phone-robot-case-v1 (Autodesk Fusion 360 design; units mm, degrees)
part number: 2026-09-02-14-29-54-371
part number: 2026-09-02-16-09-22-957
part number: 2026-09-07-14-43-40-851
part number: 2026-09-07-14-43-47-610
Autodesk Fusion 360 part; units mm, degrees
(part 1 of 2)
sketch "スケッチ1" plane through (0, 0, 0) normal (0, 0, 1) x (1, 0, 0) in component "iPhone SE 3 - Parametric Drawing Model"
  arc A0 (33.635, 60.12) -> (24.535, 69.22) centre (24.535, 60.12) ccw
  arc A1 (24.535, -69.22) -> (33.635, -60.12) centre (24.535, -60.12) ccw
  arc A2 (-33.635, -60.12) -> (-24.535, -69.22) centre (-24.535, -60.12) ccw
  arc A3 (-24.535, 69.22) -> (-33.635, 60.12) centre (-24.535, 60.12) ccw
  line L0 (-24.535, 69.22) -> (24.535, 69.22)
  line L1 (33.635, 60.12) -> (33.635, -60.12)
  line L2 (24.535, -69.22) -> (-24.535, -69.22)
  line L3 (-33.635, -60.12) -> (-33.635, 60.12)
  dimension "d710" = 49.07
  dimension "d711" = 120.24
  dimension "d712" = 9.1
  dimension "d713" = 24.535
  dimension "d714" = 60.12
  constraint horizontal L0
  constraint horizontal L2
  constraint vertical L3
  constraint vertical L1
  constraint tangent A0 L0
  constraint tangent A0 L1
  constraint tangent A1 L1
  constraint tangent A1 L2
  constraint tangent A2 L2
  constraint tangent A2 L3
  constraint tangent A3 L3
  constraint tangent A3 L0
  constraint equal A0 A1
  constraint equal A0 A2
  constraint equal A0 A3
  measures "d710" horizontal distance of A0.end A3.start
  measures "d711" vertical distance of A0.start A1.end
  measures "d712" radius of A0
  measures "d713" horizontal distance of origin A0.centre
  measures "d714" vertical distance of origin A0.centre
extrude "Rear Glass" add sketch "スケッチ1" along normal blind 0.9 makes body 1 in component "iPhone SE 3 - Parametric Drawing Model"
ref_plane "作業平面1" through (0, 0, 0.9) normal (0, 0, 1) x (1, 0, 0) in component "iPhone SE 3 - Parametric Drawing Model"
sketch "スケッチ2" plane through (0, 0, 0.9) normal (0, 0, 1) x (1, 0, 0) in component "iPhone SE 3 - Parametric Drawing Model"
  arc A0 (33.635, 60.12) -> (24.535, 69.22) centre (24.535, 60.12) ccw
  arc A1 (24.535, -69.22) -> (33.635, -60.12) centre (24.535, -60.12) ccw
  arc A2 (-33.635, -60.12) -> (-24.535, -69.22) centre (-24.535, -60.12) ccw
  arc A3 (-24.535, 69.22) -> (-33.635, 60.12) centre (-24.535, 60.12) ccw
  line L0 (-24.535, 69.22) -> (24.535, 69.22)
  line L1 (33.635, 60.12) -> (33.635, -60.12)
  line L2 (24.535, -69.22) -> (-24.535, -69.22)
  line L3 (-33.635, -60.12) -> (-33.635, 60.12)
  dimension "d719" = 49.07
  dimension "d720" = 120.24
  dimension "d721" = 9.1
  dimension "d722" = 24.535
  dimension "d723" = 60.12
  constraint horizontal L0
  constraint horizontal L2
  constraint vertical L3
  constraint vertical L1
  constraint tangent A0 L0
  constraint tangent A0 L1
  constraint tangent A1 L1
  constraint tangent A1 L2
  constraint tangent A2 L2
  constraint tangent A2 L3
  constraint tangent A3 L3
  constraint tangent A3 L0
  constraint equal A0 A1
  constraint equal A0 A2
  constraint equal A0 A3
  measures "d719" horizontal distance of A0.end A3.start
  measures "d720" vertical distance of A0.start A1.end
  measures "d721" radius of A0
  measures "d722" horizontal distance of origin A0.centre
  measures "d723" vertical distance of origin A0.centre
extrude "Aluminum Frame" add sketch "スケッチ2" along normal blind 5.51 separate body makes body 2 in component "iPhone SE 3 - Parametric Drawing Model"
ref_plane "作業平面2" through (0, 0, 6.41) normal (0, 0, 1) x (1, 0, 0) in component "iPhone SE 3 - Parametric Drawing Model"
sketch "スケッチ3" plane through (0, 0, 6.41) normal (0, 0, 1) x (1, 0, 0) in component "iPhone SE 3 - Parametric Drawing Model"
  arc A0 (33.635, 60.12) -> (24.535, 69.22) centre (24.535, 60.12) ccw
  arc A1 (24.535, -69.22) -> (33.635, -60.12) centre (24.535, -60.12) ccw
  arc A2 (-33.635, -60.12) -> (-24.535, -69.22) centre (-24.535, -60.12) ccw
  arc A3 (-24.535, 69.22) -> (-33.635, 60.12) centre (-24.535, 60.12) ccw
  line L0 (-24.535, 69.22) -> (24.535, 69.22)
  line L1 (33.635, 60.12) -> (33.635, -60.12)
  line L2 (24.535, -69.22) -> (-24.535, -69.22)
  line L3 (-33.635, -60.12) -> (-33.635, 60.12)
  dimension "d728" = 49.07
  dimension "d729" = 120.24
  dimension "d730" = 9.1
  dimension "d731" = 24.535
  dimension "d732" = 60.12
  constraint horizontal L0
  constraint horizontal L2
  constraint vertical L3
  constraint vertical L1
  constraint tangent A0 L0
  constraint tangent A0 L1
  constraint tangent A1 L1
  constraint tangent A1 L2
  constraint tangent A2 L2
  constraint tangent A2 L3
  constraint tangent A3 L3
  constraint tangent A3 L0
  constraint equal A0 A1
  constraint equal A0 A2
  constraint equal A0 A3
  measures "d728" horizontal distance of A0.end A3.start
  measures "d729" vertical distance of A0.start A1.end
  measures "d730" radius of A0
  measures "d731" horizontal distance of origin A0.centre
  measures "d732" vertical distance of origin A0.centre
extrude "Front Cover Glass" add sketch "スケッチ3" along normal blind 0.9 separate body makes body 3 in component "iPhone SE 3 - Parametric Drawing Model"
ref_plane "作業平面3" through (0, 0, 7.31) normal (0, 0, 1) x (1, 0, 0) in component "iPhone SE 3 - Parametric Drawing Model"
sketch "スケッチ4" plane through (0, 0, 7.31) normal (0, 0, 1) x (1, 0, 0) in component "iPhone SE 3 - Parametric Drawing Model"
  arc A0 (29.25, 51.23) -> (28.45, 52.03) centre (28.45, 51.23) ccw
  arc A1 (28.45, -52.02) -> (29.25, -51.22) centre (28.45, -51.22) ccw
  arc A2 (-29.25, -51.22) -> (-28.45, -52.02) centre (-28.45, -51.22) ccw
  arc A3 (-28.45, 52.03) -> (-29.25, 51.23) centre (-28.45, 51.23) ccw
  line L0 (-28.45, 52.03) -> (28.45, 52.03)
  line L1 (29.25, 51.23) -> (29.25, -51.22)
  line L2 (28.45, -52.02) -> (-28.45, -52.02)
  line L3 (-29.25, -51.22) -> (-29.25, 51.23)
  dimension "d737" = 56.9
  dimension "d738" = 102.45
  dimension "d739" = 0.8
  dimension "d740" = 28.45
  dimension "d741" = 51.23
  constraint horizontal L0
  constraint horizontal L2
  constraint vertical L3
  constraint vertical L1
  constraint tangent A0 L0
  constraint tangent A0 L1
  constraint tangent A1 L1
  constraint tangent A1 L2
  constraint tangent A2 L2
  constraint tangent A2 L3
  constraint tangent A3 L3
  constraint tangent A3 L0
  constraint equal A0 A1
  constraint equal A0 A2
  constraint equal A0 A3
  measures "d737" horizontal distance of A0.end A3.start
  measures "d738" vertical distance of A0.start A1.end
  measures "d739" radius of A0
  measures "d740" horizontal distance of origin A0.centre
  measures "d741" vertical distance of origin A0.centre
extrude "Front Active Area Reference" add sketch "スケッチ4" along normal blind 0.02 separate body makes body 4 in component "iPhone SE 3 - Parametric Drawing Model"
sketch "スケッチ5" plane through (0, 0, 7.31) normal (0, 0, 1) x (1, 0, 0) in component "iPhone SE 3 - Parametric Drawing Model"
  circle A0 centre (0, -59.97) radius 5.45
  dimension "d744" = 59.97
  dimension "d745" = 10.9
  constraint vertical origin A0.centre
  measures "d744" vertical distance of origin A0.centre
  measures "d745" diameter of A0
extrude "Home Touch ID Sensor" add sketch "スケッチ5" along normal blind 0.02 separate body makes body 5 in component "iPhone SE 3 - Parametric Drawing Model"
sketch "スケッチ6" plane through (0, 0, 7.31) normal (0, 0, 1) x (1, 0, 0) in component "iPhone SE 3 - Parametric Drawing Model"
  circle A0 centre (-10.645, 60.12) radius 1.605
  dimension "d748" = 10.645
  dimension "d749" = 60.12
  dimension "d750" = 3.21
  measures "d748" horizontal distance of origin A0.centre
  measures "d749" vertical distance of origin A0.centre
  measures "d750" diameter of A0
extrude "Front Detail 12 Front Camera Position" add sketch "スケッチ6" along normal blind 0.02 separate body makes body 6 in component "iPhone SE 3 - Parametric Drawing Model"
sketch "スケッチ7" plane through (0, 0, 7.31) normal (0, 0, 1) x (1, 0, 0) in component "iPhone SE 3 - Parametric Drawing Model"
  circle A0 centre (-0.005, 64.38) radius 1
  dimension "d753" = 0.005
  dimension "d754" = 64.38
  dimension "d755" = 2
  measures "d753" horizontal distance of origin A0.centre
  measures "d754" vertical distance of origin A0.centre
  measures "d755" diameter of A0
extrude "Front Detail 13 Proximity Sensor Position" add sketch "スケッチ7" along normal blind 0.02 separate body makes body 7 in component "iPhone SE 3 - Parametric Drawing Model"
sketch "スケッチ8" plane through (0, 0, 7.31) normal (0, 0, 1) x (1, 0, 0) in component "iPhone SE 3 - Parametric Drawing Model"
  circle A0 centre (3.685, 64.38) radius 1
  dimension "d758" = 3.685
  dimension "d759" = 64.38
  dimension "d760" = 2
  measures "d758" horizontal distance of origin A0.centre
  measures "d759" vertical distance of origin A0.centre
  measures "d760" diameter of A0
extrude "Front Detail 14 ALS Position" add sketch "スケッチ8" along normal blind 0.02 separate body makes body 8 in component "iPhone SE 3 - Parametric Drawing Model"
sketch "スケッチ9" plane through (0, 0, 7.31) normal (0, 0, 1) x (1, 0, 0) in component "iPhone SE 3 - Parametric Drawing Model"
  arc A0 (5.335, 59.52) -> (5.335, 60.72) centre (5.335, 60.12) ccw
  arc A1 (-5.335, 60.72) -> (-5.335, 59.52) centre (-5.335, 60.12) ccw
  line L0 (-5.335, 60.72) -> (5.335, 60.72)
  line L1 (5.335, 59.52) -> (-5.335, 59.52)
  line L2 (-5.335, 60.12) -> (5.335, 60.12) construction
  point P0 (0, 60.12)
  dimension "d763" = 10.67
  dimension "d764" = 0.6
  dimension "d765" = 60.12
  constraint horizontal L0
  constraint horizontal L1
  constraint equal A0 A1
  constraint midpoint L2 P0
  constraint vertical origin P0
  measures "d763" horizontal distance of A0.centre A1.centre
  measures "d764" radius of A0
  measures "d765" vertical distance of origin P0
extrude "Receiver Opening" add sketch "スケッチ9" along normal blind 0.02 separate body makes body 9 in component "iPhone SE 3 - Parametric Drawing Model"
sketch "スケッチ10" plane through (0, 0, 0) normal (0, 0, 1) x (1, 0, 0) in component "iPhone SE 3 - Parametric Drawing Model"
  circle A0 centre (-23.195, 53.82) radius 4.285
  dimension "d768" = 23.195
  dimension "d769" = 53.82
  dimension "d770" = 8.57
  measures "d768" horizontal distance of origin A0.centre
  measures "d769" vertical distance of origin A0.centre
  measures "d770" diameter of A0
extrude "Rear Camera Bump" add sketch "スケッチ10" against normal blind 0.87 separate body makes body 10 in component "iPhone SE 3 - Parametric Drawing Model"
sketch "スケッチ11" plane through (0, 0, 0) normal (0, 0, 1) x (1, 0, 0) in component "iPhone SE 3 - Parametric Drawing Model"
  circle A0 centre (-15.505, 53.82) radius 0.75
  dimension "d773" = 15.505
  dimension "d774" = 53.82
  dimension "d775" = 1.5
  measures "d773" horizontal distance of origin A0.centre
  measures "d774" vertical distance of origin A0.centre
  measures "d775" diameter of A0
extrude "Rear Microphone" add sketch "スケッチ11" against normal blind 0.02 separate body makes body 11 in component "iPhone SE 3 - Parametric Drawing Model"
sketch "スケッチ12" plane through (0, 0, 0) normal (0, 0, 1) x (1, 0, 0) in component "iPhone SE 3 - Parametric Drawing Model"
  circle A0 centre (-10.795, 53.82) radius 1.875
  dimension "d778" = 10.795
  dimension "d779" = 53.82
  dimension "d780" = 3.75
  measures "d778" horizontal distance of origin A0.centre
  measures "d779" vertical distance of origin A0.centre
  measures "d780" diameter of A0
extrude "Rear Flash" add sketch "スケッチ12" against normal blind 0.02 separate body makes body 12 in component "iPhone SE 3 - Parametric Drawing Model"
ref_plane "作業平面4" through (-33.635, 0, 0) normal (1, 0, 0) x (0, 1, 0) in component "iPhone SE 3 - Parametric Drawing Model"
ref_plane "作業平面5" through (33.635, 0, 0) normal (1, 0, 0) x (0, 1, 0) in component "iPhone SE 3 - Parametric Drawing Model"
sketch "スケッチ13" plane through (-33.635, 0, 0) normal (1, 0, 0) x (0, 0, -1) in component "iPhone SE 3 - Parametric Drawing Model"
  arc A0 (-2.755, 50.76) -> (-4.555, 50.76) centre (-3.655, 50.76) ccw
  arc A1 (-4.555, 46.95) -> (-2.755, 46.95) centre (-3.655, 46.95) ccw
  line L0 (-2.755, 50.76) -> (-2.755, 46.95)
  line L1 (-4.555, 46.95) -> (-4.555, 50.76)
  line L2 (-3.655, 50.76) -> (-3.655, 46.95) construction
  point P0 (-3.655, 48.855)
  dimension "d787" = 3.81
  dimension "d788" = 0.9
  dimension "d789" = 3.655
  dimension "d790" = 48.855
  constraint vertical L0
  constraint vertical L1
  constraint equal A0 A1
  constraint midpoint L2 P0
  measures "d787" vertical distance of A0.centre A1.centre
  measures "d788" radius of A0
  measures "d789" horizontal distance of origin P0
  measures "d790" vertical distance of origin P0
extrude "Ring Silent Switch" add sketch "スケッチ13" against normal blind 0.42 separate body makes body 13 in component "iPhone SE 3 - Parametric Drawing Model"
sketch "スケッチ14" plane through (-33.635, 0, 0) normal (1, 0, 0) x (0, 0, -1) in component "iPhone SE 3 - Parametric Drawing Model"
  arc A0 (-2.755, 39.07) -> (-4.555, 39.07) centre (-3.655, 39.07) ccw
  arc A1 (-4.555, 30.25) -> (-2.755, 30.25) centre (-3.655, 30.25) ccw
  line L0 (-2.755, 39.07) -> (-2.755, 30.25)
  line L1 (-4.555, 30.25) -> (-4.555, 39.07)
  line L2 (-3.655, 39.07) -> (-3.655, 30.25) construction
  point P0 (-3.655, 34.66)
  dimension "d793" = 8.82
  dimension "d794" = 0.9
  dimension "d795" = 3.655
  dimension "d796" = 34.66
  constraint vertical L0
  constraint vertical L1
  constraint equal A0 A1
  constraint midpoint L2 P0
  measures "d793" vertical distance of A0.centre A1.centre
  measures "d794" radius of A0
  measures "d795" horizontal distance of origin P0
  measures "d796" vertical distance of origin P0
extrude "Volume Plus Button" add sketch "スケッチ14" against normal blind 0.4 separate body makes body 14 in component "iPhone SE 3 - Parametric Drawing Model"
sketch "スケッチ15" plane through (-33.635, 0, 0) normal (1, 0, 0) x (0, 0, -1) in component "iPhone SE 3 - Parametric Drawing Model"
  arc A0 (-2.755, 26.46) -> (-4.555, 26.46) centre (-3.655, 26.46) ccw
  arc A1 (-4.555, 17.64) -> (-2.755, 17.64) centre (-3.655, 17.64) ccw
  line L0 (-2.755, 26.46) -> (-2.755, 17.64)
  line L1 (-4.555, 17.64) -> (-4.555, 26.46)
  line L2 (-3.655, 26.46) -> (-3.655, 17.64) construction
  point P0 (-3.655, 22.05)
  dimension "d799" = 8.82
  dimension "d800" = 0.9
  dimension "d801" = 3.655
  dimension "d802" = 22.05
  constraint vertical L0
  constraint vertical L1
  constraint equal A0 A1
  constraint midpoint L2 P0
  measures "d799" vertical distance of A0.centre A1.centre
  measures "d800" radius of A0
  measures "d801" horizontal distance of origin P0
  measures "d802" vertical distance of origin P0
extrude "Volume Minus Button" add sketch "スケッチ15" against normal blind 0.4 separate body makes body 15 in component "iPhone SE 3 - Parametric Drawing Model"
sketch "スケッチ16" plane through (33.635, 0, 0) normal (1, 0, 0) x (0, 0, -1) in component "iPhone SE 3 - Parametric Drawing Model"
  arc A0 (-2.755, 38.99) -> (-4.555, 38.99) centre (-3.655, 38.99) ccw
  arc A1 (-4.555, 30.17) -> (-2.755, 30.17) centre (-3.655, 30.17) ccw
  line L0 (-2.755, 38.99) -> (-2.755, 30.17)
  line L1 (-4.555, 30.17) -> (-4.555, 38.99)
  line L2 (-3.655, 38.99) -> (-3.655, 30.17) construction
  point P0 (-3.655, 34.58)
  dimension "d805" = 8.82
  dimension "d806" = 0.9
  dimension "d807" = 3.655
  dimension "d808" = 34.58
  constraint vertical L0
  constraint vertical L1
  constraint equal A0 A1
  constraint midpoint L2 P0
  measures "d805" vertical distance of A0.centre A1.centre
  measures "d806" radius of A0
  measures "d807" horizontal distance of origin P0
  measures "d808" vertical distance of origin P0
extrude "Side Button" add sketch "スケッチ16" along normal blind 0.4 separate body makes body 16 in component "iPhone SE 3 - Parametric Drawing Model"
sketch "スケッチ17" plane through (33.635, 0, 0) normal (1, 0, 0) x (0, 0, -1) in component "iPhone SE 3 - Parametric Drawing Model"
  arc A0 (-2.505, 15.35) -> (-4.805, 15.35) centre (-3.655, 15.35) ccw
  arc A1 (-4.805, 1.98) -> (-2.505, 1.98) centre (-3.655, 1.98) ccw
  line L0 (-2.505, 15.35) -> (-2.505, 1.98)
  line L1 (-4.805, 1.98) -> (-4.805, 15.35)
  line L2 (-3.655, 15.35) -> (-3.655, 1.98) construction
  point P0 (-3.655, 8.665)
  dimension "d811" = 13.37
  dimension "d812" = 1.15
  dimension "d813" = 3.655
  dimension "d814" = 8.665
  constraint vertical L0
  constraint vertical L1
  constraint equal A0 A1
  constraint midpoint L2 P0
  measures "d811" vertical distance of A0.centre A1.centre
  measures "d812" radius of A0
  measures "d813" horizontal distance of origin P0
  measures "d814" vertical distance of origin P0
extrude "SIM Tray Seam" cut sketch "スケッチ17" against normal blind 0.05 bodies 2 in component "iPhone SE 3 - Parametric Drawing Model"
ref_plane "作業平面6" through (0, -69.22, 0) normal (0, 1, 0) x (0, 0, 1) in component "iPhone SE 3 - Parametric Drawing Model"
sketch "スケッチ18" plane through (0, -69.22, 0) normal (0, 1, 0) x (1, 0, 0) in component "iPhone SE 3 - Parametric Drawing Model"
  arc A0 (3.55, -4.455) -> (3.55, -2.855) centre (3.55, -3.655) ccw
  arc A1 (-3.55, -2.855) -> (-3.55, -4.455) centre (-3.55, -3.655) ccw
  line L0 (-3.55, -2.855) -> (3.55, -2.855)
  line L1 (3.55, -4.455) -> (-3.55, -4.455)
  line L2 (-3.55, -3.655) -> (3.55, -3.655) construction
  circle A2 centre (-23.375, -3.655) radius 0.725
  circle A3 centre (-20.975, -3.655) radius 0.725
  circle A4 centre (-18.575, -3.655) radius 0.725
  circle A5 centre (-16.175, -3.655) radius 0.725
  circle A6 centre (-13.775, -3.655) radius 0.725
  circle A7 centre (-11.375, -3.655) radius 0.725
  circle A8 centre (11.375, -3.655) radius 0.725
  circle A9 centre (13.775, -3.655) radius 0.725
  circle A10 centre (16.175, -3.655) radius 0.725
  circle A11 centre (18.575, -3.655) radius 0.725
  circle A12 centre (20.975, -3.655) radius 0.725
  circle A13 centre (23.375, -3.655) radius 0.725
  circle A14 centre (-6.395, -3.655) radius 0.8
  circle A15 centre (6.395, -3.655) radius 0.8
  point P0 (0, -3.655)
  dimension "d819" = 7.1
  dimension "d820" = 0.8
  dimension "d821" = 3.655
  dimension "d822" = 23.375
  dimension "d823" = 3.655
  dimension "d824" = 1.45
  dimension "d825" = 20.975
  dimension "d826" = 3.655
  dimension "d827" = 1.45
  dimension "d828" = 18.575
  dimension "d829" = 3.655
  dimension "d830" = 1.45
  dimension "d831" = 16.175
  dimension "d832" = 3.655
  dimension "d833" = 1.45
  dimension "d834" = 13.775
  dimension "d835" = 3.655
  dimension "d836" = 1.45
  dimension "d837" = 11.375
  dimension "d838" = 3.655
  dimension "d839" = 1.45
  dimension "d840" = 11.375
  dimension "d841" = 3.655
  dimension "d842" = 1.45
  dimension "d843" = 13.775
  dimension "d844" = 3.655
  dimension "d845" = 1.45
  dimension "d846" = 16.175
  dimension "d847" = 3.655
  dimension "d848" = 1.45
  dimension "d849" = 18.575
  dimension "d850" = 3.655
  dimension "d851" = 1.45
  dimension "d852" = 20.975
  dimension "d853" = 3.655
  dimension "d854" = 1.45
  dimension "d855" = 23.375
  dimension "d856" = 3.655
  dimension "d857" = 1.45
  dimension "d858" = 6.395
  dimension "d859" = 3.655
  dimension "d860" = 1.6
  dimension "d861" = 6.395
  dimension "d862" = 3.655
  dimension "d863" = 1.6
  constraint horizontal L0
  constraint horizontal L1
  constraint equal A0 A1
  constraint midpoint L2 P0
  constraint vertical origin P0
  measures "d819" horizontal distance of A0.centre A1.centre
  measures "d820" radius of A0
  measures "d821" vertical distance of origin P0
  measures "d822" horizontal distance of origin A2.centre
  measures "d823" vertical distance of origin A2.centre
  measures "d824" diameter of A2
  measures "d825" horizontal distance of origin A3.centre
  measures "d826" vertical distance of origin A3.centre
  measures "d827" diameter of A3
  measures "d828" horizontal distance of origin A4.centre
  measures "d829" vertical distance of origin A4.centre
  measures "d830" diameter of A4
  measures "d831" horizontal distance of origin A5.centre
  measures "d832" vertical distance of origin A5.centre
  measures "d833" diameter of A5
  measures "d834" horizontal distance of origin A6.centre
  measures "d835" vertical distance of origin A6.centre
  measures "d836" diameter of A6
  measures "d837" horizontal distance of origin A7.centre
  measures "d838" vertical distance of origin A7.centre
  measures "d839" diameter of A7
  measures "d840" horizontal distance of origin A8.centre
  measures "d841" vertical distance of origin A8.centre
  measures "d842" diameter of A8
  measures "d843" horizontal distance of origin A9.centre
  measures "d844" vertical distance of origin A9.centre
  measures "d845" diameter of A9
  measures "d846" horizontal distance of origin A10.centre
  measures "d847" vertical distance of origin A10.centre
  measures "d848" diameter of A10
  measures "d849" horizontal distance of origin A11.centre
  measures "d850" vertical distance of origin A11.centre
  measures "d851" diameter of A11
  measures "d852" horizontal distance of origin A12.centre
  measures "d853" vertical distance of origin A12.centre
  measures "d854" diameter of A12
  measures "d855" horizontal distance of origin A13.centre
  measures "d856" vertical distance of origin A13.centre
  measures "d857" diameter of A13
  measures "d858" horizontal distance of origin A14.centre
  measures "d859" vertical distance of origin A14.centre
  measures "d860" diameter of A14
  measures "d861" horizontal distance of origin A15.centre
  measures "d862" vertical distance of origin A15.centre
  measures "d863" diameter of A15
extrude "Bottom Port and Acoustic Openings" cut sketch "スケッチ18" along normal blind 1 bodies 2 in component "iPhone SE 3 - Parametric Drawing Model"
ref_plane "作業平面7" through (0, 0, 3.655) normal (0, 0, 1) x (1, 0, 0) in component "iPhone SE 3 - Parametric Drawing Model"
sketch "スケッチ19" plane through (0, 0, 3.655) normal (0, 0, 1) x (1, 0, 0) in component "iPhone SE 3 - Parametric Drawing Model"
  arc A0 (33.635, 60.12) -> (24.535, 69.22) centre (24.535, 60.12) ccw
  arc A1 (24.535, -69.22) -> (33.635, -60.12) centre (24.535, -60.12) ccw
  arc A2 (-33.635, -60.12) -> (-24.535, -69.22) centre (-24.535, -60.12) ccw
  arc A3 (-24.535, 69.22) -> (-33.635, 60.12) centre (-24.535, 60.12) ccw
  line L0 (-24.535, 69.22) -> (24.535, 69.22)
  line L1 (33.635, 60.12) -> (33.635, -60.12)
  line L2 (24.535, -69.22) -> (-24.535, -69.22)
  line L3 (-33.635, -60.12) -> (-33.635, 60.12)
  dimension "d868" = 49.07
  dimension "d869" = 120.24
  dimension "d870" = 9.1
  dimension "d871" = 24.535
  dimension "d872" = 60.12
  constraint horizontal L0
  constraint horizontal L2
  constraint vertical L3
  constraint vertical L1
  constraint tangent A0 L0
  constraint tangent A0 L1
  constraint tangent A1 L1
  constraint tangent A1 L2
  constraint tangent A2 L2
  constraint tangent A2 L3
  constraint tangent A3 L3
  constraint tangent A3 L0
  constraint equal A0 A1
  constraint equal A0 A2
  constraint equal A0 A3
  measures "d868" horizontal distance of A0.end A3.start
  measures "d869" vertical distance of A0.start A1.end
  measures "d870" radius of A0
  measures "d871" horizontal distance of origin A0.centre
  measures "d872" vertical distance of origin A0.centre
ref_plane "作業平面1" through (0, 0, -2.9) normal (0, 0, 1) x (1, 0, 0) in component "Robot V1 - A Holder and Stand"
ref_plane "作業平面2" through (0, 0, -0.5) normal (0, 0, 1) x (1, 0, 0) in component "Robot V1 - A Holder and Stand"
ref_plane "作業平面3" through (0, 0, 7.71) normal (0, 0, 1) x (1, 0, 0) in component "Robot V1 - A Holder and Stand"
sketch "スケッチ1 (2)" plane through (0, 0, -2.9) normal (0, 0, 1) x (1, 0, 0) in component "Robot V1 - A Holder and Stand"
  arc A0 (46, 68) -> (40, 74) centre (40, 68) ccw
  arc A1 (40, 14) -> (46, 20) centre (40, 20) ccw
  arc A2 (-46, 20) -> (-40, 14) centre (-40, 20) ccw
  arc A3 (-40, 74) -> (-46, 68) centre (-40, 68) ccw
  line L0 (-40, 74) -> (40, 74)
  line L1 (46, 68) -> (46, 20)
  line L2 (40, 14) -> (-40, 14)
  line L3 (-46, 20) -> (-46, 68)
  line L4 (40, 68) -> (-40, 20) construction
  point P0 (0, 44)
  dimension "d1520" = 80
  dimension "d1521" = 48
  dimension "d1522" = 6
  dimension "d1523" = 44
  constraint horizontal L0
  constraint horizontal L2
  constraint vertical L3
  constraint vertical L1
  constraint tangent A0 L0
  constraint tangent A0 L1
  constraint tangent A1 L1
  constraint tangent A1 L2
  constraint tangent A2 L2
  constraint tangent A2 L3
  constraint tangent A3 L3
  constraint tangent A3 L0
  constraint equal A0 A1
  constraint equal A0 A2
  constraint equal A0 A3
  constraint midpoint L4 P0
  constraint vertical origin P0
  measures "d1520" horizontal distance of A0.end A3.start
  measures "d1521" vertical distance of A0.start A1.end
  measures "d1522" radius of A0
  measures "d1523" vertical distance of origin P0
extrude "A 01 Head plate" add sketch "スケッチ1 (2)" along normal blind 2.4 separate body makes body 17 in component "Robot V1 - A Holder and Stand"
sketch "スケッチ2 (2)" plane through (0, 0, -2.9) normal (0, 0, 1) x (1, 0, 0) in component "Robot V1 - A Holder and Stand"
  arc A0 (41, 16) -> (35, 22) centre (35, 16) ccw
  arc A1 (35, -74) -> (41, -68) centre (35, -68) ccw
  arc A2 (-41, -68) -> (-35, -74) centre (-35, -68) ccw
  arc A3 (-35, 22) -> (-41, 16) centre (-35, 16) ccw
  line L0 (-35, 22) -> (35, 22)
  line L1 (41, 16) -> (41, -68)
  line L2 (35, -74) -> (-35, -74)
  line L3 (-41, -68) -> (-41, 16)
  line L4 (35, 16) -> (-35, -68) construction
  point P0 (0, -26)
  dimension "d1526" = 70
  dimension "d1527" = 84
  dimension "d1528" = 6
  dimension "d1529" = 26
  constraint horizontal L0
  constraint horizontal L2
  constraint vertical L3
  constraint vertical L1
  constraint tangent A0 L0
  constraint tangent A0 L1
  constraint tangent A1 L1
  constraint tangent A1 L2
  constraint tangent A2 L2
  constraint tangent A2 L3
  constraint tangent A3 L3
  constraint tangent A3 L0
  constraint equal A0 A1
  constraint equal A0 A2
  constraint equal A0 A3
  constraint midpoint L4 P0
  constraint vertical origin P0
  measures "d1526" horizontal distance of A0.end A3.start
  measures "d1527" vertical distance of A0.start A1.end
  measures "d1528" radius of A0
  measures "d1529" vertical distance of origin P0
extrude "A 02 Body plate" add sketch "スケッチ2 (2)" along normal blind 2.4 bodies 17 in component "Robot V1 - A Holder and Stand"
sketch "スケッチ3 (2)" plane through (0, 0, -0.5) normal (0, 0, 1) x (1, 0, 0) in component "Robot V1 - A Holder and Stand"
  arc A0 (36.435, 60.12) -> (24.535, 72.02) centre (24.535, 60.12) ccw
  arc A1 (24.535, -72.02) -> (36.435, -60.12) centre (24.535, -60.12) ccw
  arc A2 (-36.435, -60.12) -> (-24.535, -72.02) centre (-24.535, -60.12) ccw
  arc A3 (-24.535, 72.02) -> (-36.435, 60.12) centre (-24.535, 60.12) ccw
  line L0 (-24.535, 72.02) -> (24.535, 72.02)
  line L1 (36.435, 60.12) -> (36.435, -60.12)
  line L2 (24.535, -72.02) -> (-24.535, -72.02)
  line L3 (-36.435, -60.12) -> (-36.435, 60.12)
  line L4 (24.535, 60.12) -> (-24.535, -60.12) construction
  dimension "d1532" = 49.07
  dimension "d1533" = 120.24
  dimension "d1534" = 11.9
  constraint horizontal L0
  constraint horizontal L2
  constraint vertical L3
  constraint vertical L1
  constraint tangent A0 L0
  constraint tangent A0 L1
  constraint tangent A1 L1
  constraint tangent A1 L2
  constraint tangent A2 L2
  constraint tangent A2 L3
  constraint tangent A3 L3
  constraint tangent A3 L0
  constraint equal A0 A1
  constraint equal A0 A2
  constraint equal A0 A3
  constraint midpoint L4 origin
  measures "d1532" horizontal distance of A0.end A3.start
  measures "d1533" vertical distance of A0.start A1.end
  measures "d1534" radius of A0
extrude "A03 Tray wall blank" add sketch "スケッチ3 (2)" along normal blind 8.21 bodies 17 in component "Robot V1 - A Holder and Stand"
sketch "スケッチ4 (2)" plane through (0, 0, -0.5) normal (0, 0, 1) x (1, 0, 0) in component "Robot V1 - A Holder and Stand"
  circle A0 centre (-40, 62) radius 5
  dimension "d1537" = 40
  dimension "d1538" = 62
  dimension "d1539" = 10
  measures "d1537" horizontal distance of origin A0.centre
  measures "d1538" vertical distance of origin A0.centre
  measures "d1539" diameter of A0
extrude "A04 TL pad" add sketch "スケッチ4 (2)" along normal blind 8.21 bodies 17 in component "Robot V1 - A Holder and Stand"
sketch "スケッチ5 (2)" plane through (0, 0, -0.5) normal (0, 0, 1) x (1, 0, 0) in component "Robot V1 - A Holder and Stand"
  circle A0 centre (40, 62) radius 5
  dimension "d1542" = 40
  dimension "d1543" = 62
  dimension "d1544" = 10
  measures "d1542" horizontal distance of origin A0.centre
  measures "d1543" vertical distance of origin A0.centre
  measures "d1544" diameter of A0
extrude "A04 TR pad" add sketch "スケッチ5 (2)" along normal blind 8.21 bodies 17 in component "Robot V1 - A Holder and Stand"
sketch "スケッチ6 (2)" plane through (0, 0, -0.5) normal (0, 0, 1) x (1, 0, 0) in component "Robot V1 - A Holder and Stand"
  circle A0 centre (-37, -62) radius 4
  dimension "d1547" = 37
  dimension "d1548" = 62
  dimension "d1549" = 8
  measures "d1547" horizontal distance of origin A0.centre
  measures "d1548" vertical distance of origin A0.centre
  measures "d1549" diameter of A0
extrude "A04 BL pad" add sketch "スケッチ6 (2)" along normal blind 8.21 bodies 17 in component "Robot V1 - A Holder and Stand"
sketch "スケッチ7 (2)" plane through (0, 0, -0.5) normal (0, 0, 1) x (1, 0, 0) in component "Robot V1 - A Holder and Stand"
  circle A0 centre (37, -62) radius 4
  dimension "d1552" = 37
  dimension "d1553" = 62
  dimension "d1554" = 8
  measures "d1552" horizontal distance of origin A0.centre
  measures "d1553" vertical distance of origin A0.centre
  measures "d1554" diameter of A0
extrude "A04 BR pad" add sketch "スケッチ7 (2)" along normal blind 8.21 bodies 17 in component "Robot V1 - A Holder and Stand"
sketch "スケッチ8 (2)" plane through (0, 0, 7.71) normal (0, 0, 1) x (1, 0, 0) in component "Robot V1 - A Holder and Stand"
  arc A0 (34.035, 60.12) -> (24.535, 69.62) centre (24.535, 60.12) ccw
  arc A1 (24.535, -69.62) -> (34.035, -60.12) centre (24.535, -60.12) ccw
  arc A2 (-34.035, -60.12) -> (-24.535, -69.62) centre (-24.535, -60.12) ccw
  arc A3 (-24.535, 69.62) -> (-34.035, 60.12) centre (-24.535, 60.12) ccw
  line L0 (-24.535, 69.62) -> (24.535, 69.62)
  line L1 (34.035, 60.12) -> (34.035, -60.12)
  line L2 (24.535, -69.62) -> (-24.535, -69.62)
  line L3 (-34.035, -60.12) -> (-34.035, 60.12)
  line L4 (24.535, 60.12) -> (-24.535, -60.12) construction
  dimension "d1557" = 49.07
  dimension "d1558" = 120.24
  dimension "d1559" = 9.5
  constraint horizontal L0
  constraint horizontal L2
  constraint vertical L3
  constraint vertical L1
  constraint tangent A0 L0
  constraint tangent A0 L1
  constraint tangent A1 L1
  constraint tangent A1 L2
  constraint tangent A2 L2
  constraint tangent A2 L3
  constraint tangent A3 L3
  constraint tangent A3 L0
  constraint equal A0 A1
  constraint equal A0 A2
  constraint equal A0 A3
  constraint midpoint L4 origin
  measures "d1557" horizontal distance of A0.end A3.start
  measures "d1558" vertical distance of A0.start A1.end
  measures "d1559" radius of A0
extrude "A05 Phone pocket" cut sketch "スケッチ8 (2)" against normal blind 8.21 bodies 17 in component "Robot V1 - A Holder and Stand"
sketch "スケッチ9 (2)" plane through (0, 0, 7.71) normal (0, 0, 1) x (1, 0, 0) in component "Robot V1 - A Holder and Stand"
  line L0 (-30.435, 58) -> (-42.435, 58)
  line L1 (-42.435, 58) -> (-42.435, 10)
  line L2 (-42.435, 10) -> (-30.435, 10)
  line L3 (-30.435, 10) -> (-30.435, 58)
  line L4 (-30.435, 58) -> (-42.435, 10) construction
  point P0 (-36.435, 34)
  dimension "d1562" = 36.435
  dimension "d1563" = 34
  dimension "d1564" = 12
  dimension "d1565" = 48
  constraint horizontal L0
  constraint vertical L1
  constraint horizontal L2
  constraint vertical L3
  constraint midpoint L4 P0
  measures "d1562" horizontal distance of origin P0
  measures "d1563" vertical distance of origin P0
  measures "d1564" horizontal distance of L0.start L0.end
  measures "d1565" vertical distance of L0.end L1.end
extrude "A06 Left side opening" cut sketch "スケッチ9 (2)" against normal blind 8.21 bodies 17 in component "Robot V1 - A Holder and Stand"
sketch "スケッチ10 (2)" plane through (0, 0, 7.71) normal (0, 0, 1) x (1, 0, 0) in component "Robot V1 - A Holder and Stand"
  line L0 (42.435, 58) -> (30.435, 58)
  line L1 (30.435, 58) -> (30.435, 10)
  line L2 (30.435, 10) -> (42.435, 10)
  line L3 (42.435, 10) -> (42.435, 58)
  line L4 (42.435, 58) -> (30.435, 10) construction
  point P0 (36.435, 34)
  dimension "d1568" = 36.435
  dimension "d1569" = 34
  dimension "d1570" = 12
  dimension "d1571" = 48
  constraint horizontal L0
  constraint vertical L1
  constraint horizontal L2
  constraint vertical L3
  constraint midpoint L4 P0
  measures "d1568" horizontal distance of origin P0
  measures "d1569" vertical distance of origin P0
  measures "d1570" horizontal distance of L0.start L0.end
  measures "d1571" vertical distance of L0.end L1.end
extrude "A06 Right side opening" cut sketch "スケッチ10 (2)" against normal blind 8.21 bodies 17 in component "Robot V1 - A Holder and Stand"
sketch "スケッチ11 (2)" plane through (0, 0, 7.71) normal (0, 0, 1) x (1, 0, 0) in component "Robot V1 - A Holder and Stand"
  line L0 (27, -66) -> (-27, -66)
  line L1 (-27, -66) -> (-27, -82)
  line L2 (-27, -82) -> (27, -82)
  line L3 (27, -82) -> (27, -66)
  line L4 (27, -66) -> (-27, -82) construction
  point P0 (0, -74)
  dimension "d1574" = 74
  dimension "d1575" = 54
  dimension "d1576" = 16
  constraint horizontal L0
  constraint vertical L1
  constraint horizontal L2
  constraint vertical L3
  constraint midpoint L4 P0
  constraint vertical origin P0
  measures "d1574" vertical distance of origin P0
  measures "d1575" horizontal distance of L0.start L0.end
  measures "d1576" vertical distance of L0.end L1.end
extrude "A07 Open bottom" cut sketch "スケッチ11 (2)" against normal blind 10.61 bodies 17 in component "Robot V1 - A Holder and Stand"
sketch "スケッチ12 (2)" plane through (0, 0, 7.71) normal (0, 0, 1) x (1, 0, 0) in component "Robot V1 - A Holder and Stand"
  arc A0 (-5, 61.5) -> (-7, 63.5) centre (-7, 61.5) ccw
  arc A1 (-7, 45.5) -> (-5, 47.5) centre (-7, 47.5) ccw
  arc A2 (-31, 47.5) -> (-29, 45.5) centre (-29, 47.5) ccw
  arc A3 (-29, 63.5) -> (-31, 61.5) centre (-29, 61.5) ccw
  line L0 (-29, 63.5) -> (-7, 63.5)
  line L1 (-5, 61.5) -> (-5, 47.5)
  line L2 (-7, 45.5) -> (-29, 45.5)
  line L3 (-31, 47.5) -> (-31, 61.5)
  line L4 (-7, 61.5) -> (-29, 47.5) construction
  point P0 (-18, 54.5)
  dimension "d1579" = 22
  dimension "d1580" = 14
  dimension "d1581" = 2
  dimension "d1582" = 18
  dimension "d1583" = 54.5
  constraint horizontal L0
  constraint horizontal L2
  constraint vertical L3
  constraint vertical L1
  constraint tangent A0 L0
  constraint tangent A0 L1
  constraint tangent A1 L1
  constraint tangent A1 L2
  constraint tangent A2 L2
  constraint tangent A2 L3
  constraint tangent A3 L3
  constraint tangent A3 L0
  constraint equal A0 A1
  constraint equal A0 A2
  constraint equal A0 A3
  constraint midpoint L4 P0
  measures "d1579" horizontal distance of A0.end A3.start
  measures "d1580" vertical distance of A0.start A1.end
  measures "d1581" radius of A0
  measures "d1582" horizontal distance of origin P0
  measures "d1583" vertical distance of origin P0
extrude "A08 Rear camera opening" cut sketch "スケッチ12 (2)" against normal blind 10.61 bodies 17 in component "Robot V1 - A Holder and Stand"
sketch "スケッチ13 (2)" plane through (0, 0, 7.71) normal (0, 0, 1) x (1, 0, 0) in component "Robot V1 - A Holder and Stand"
  arc A0 (20, 20) -> (16, 24) centre (16, 20) ccw
  arc A1 (16, -38) -> (20, -34) centre (16, -34) ccw
  arc A2 (-20, -34) -> (-16, -38) centre (-16, -34) ccw
  arc A3 (-16, 24) -> (-20, 20) centre (-16, 20) ccw
  line L0 (-16, 24) -> (16, 24)
  line L1 (20, 20) -> (20, -34)
  line L2 (16, -38) -> (-16, -38)
  line L3 (-20, -34) -> (-20, 20)
  line L4 (16, 20) -> (-16, -34) construction
  point P0 (0, -7)
  dimension "d1586" = 32
  dimension "d1587" = 54
  dimension "d1588" = 4
  dimension "d1589" = 7
  constraint horizontal L0
  constraint horizontal L2
  constraint vertical L3
  constraint vertical L1
  constraint tangent A0 L0
  constraint tangent A0 L1
  constraint tangent A1 L1
  constraint tangent A1 L2
  constraint tangent A2 L2
  constraint tangent A2 L3
  constraint tangent A3 L3
  constraint tangent A3 L0
  constraint equal A0 A1
  constraint equal A0 A2
  constraint equal A0 A3
  constraint midpoint L4 P0
  constraint vertical origin P0
  measures "d1586" horizontal distance of A0.end A3.start
  measures "d1587" vertical distance of A0.start A1.end
  measures "d1588" radius of A0
  measures "d1589" vertical distance of origin P0
extrude "A09 Rear ventilation" cut sketch "スケッチ13 (2)" against normal blind 10.61 bodies 17 in component "Robot V1 - A Holder and Stand"
ref_plane "作業平面4" through (-31, 0, 0) normal (1, 0, 0) x (0, 1, 0) in component "Robot V1 - A Holder and Stand"
sketch "スケッチ15 (2)" plane through (-31, 0, 0) normal (1, 0, 0) x (0, 0, -1) in component "Robot V1 - A Holder and Stand"
  line L0 (0.5, 0) -> (0.5, -101.1063)
  line L1 (0.5, -101.1063) -> (64.5577, -87.4904)
  line L2 (64.5577, -87.4904) -> (0.5, 0)
  dimension "d1594" = 0.5
  dimension "d1595" = 101.1063
  dimension "d1596" = 64.5577
  dimension "d1597" = 87.4904
  constraint horizontal origin L0.start
  constraint vertical L0.start L0.end
  measures "d1594" horizontal distance of origin L0.start
  measures "d1595" vertical distance of origin L0.end
  measures "d1596" horizontal distance of origin L1.end
  measures "d1597" vertical distance of origin L1.end
extrude "A10 L rear stand rib" add sketch "スケッチ15 (2)" along normal blind 4 bodies 17 in component "Robot V1 - A Holder and Stand"
ref_plane "作業平面5" through (27, 0, 0) normal (1, 0, 0) x (0, 1, 0) in component "Robot V1 - A Holder and Stand"
sketch "スケッチ16 (2)" plane through (27, 0, 0) normal (1, 0, 0) x (0, 0, -1) in component "Robot V1 - A Holder and Stand"
  line L0 (0.5, 0) -> (0.5, -101.1063)
  line L1 (0.5, -101.1063) -> (64.5577, -87.4904)
  line L2 (64.5577, -87.4904) -> (0.5, 0)
  dimension "d1602" = 0.5
  dimension "d1603" = 101.1063
  dimension "d1604" = 64.5577
  dimension "d1605" = 87.4904
  constraint horizontal origin L0.start
  constraint vertical L0.start L0.end
  measures "d1602" horizontal distance of origin L0.start
  measures "d1603" vertical distance of origin L0.end
  measures "d1604" horizontal distance of origin L1.end
  measures "d1605" vertical distance of origin L1.end
extrude "A10 R rear stand rib" add sketch "スケッチ16 (2)" along normal blind 4 bodies 17 in component "Robot V1 - A Holder and Stand"
ref_plane "作業平面6" through (-50, 0, 0) normal (1, 0, 0) x (0, 1, 0) in component "Robot V1 - A Holder and Stand"
sketch "スケッチ17 (2)" plane through (-50, 0, 0) normal (1, 0, 0) x (0, 0, -1) in component "Robot V1 - A Holder and Stand"
  line L0 (-19.563, -109.1602) -> (68.4703, -90.4481)
  line L1 (68.4703, -90.4481) -> (67.6387, -86.5355)
  line L2 (67.6387, -86.5355) -> (-20.3946, -105.2476)
  line L3 (-20.3946, -105.2476) -> (-19.563, -109.1602)
  dimension "d1610" = 19.563
  dimension "d1611" = 109.1602
  dimension "d1612" = 68.4703
  dimension "d1613" = 90.4481
  dimension "d1614" = 67.6387
  dimension "d1615" = 86.5355
  dimension "d1616" = 20.3946
  dimension "d1617" = 105.2476
  measures "d1610" horizontal distance of origin L0.start
  measures "d1611" vertical distance of origin L0.start
  measures "d1612" horizontal distance of origin L0.end
  measures "d1613" vertical distance of origin L0.end
  measures "d1614" horizontal distance of origin L1.end
  measures "d1615" vertical distance of origin L1.end
  measures "d1616" horizontal distance of origin L2.end
  measures "d1617" vertical distance of origin L2.end
extrude "A11 Desk base" add sketch "スケッチ17 (2)" along normal blind 100 bodies 17 in component "Robot V1 - A Holder and Stand"
ref_plane "作業平面7" through (0, 0, 4) normal (0, 0, 1) x (1, 0, 0) in component "Robot V1 - A Holder and Stand"
sketch "スケッチ18 (2)" plane through (0, 0, 4) normal (0, 0, 1) x (1, 0, 0) in component "Robot V1 - A Holder and Stand"
  line L0 (8, -60.0019) -> (-8, -60.0019)
  line L1 (-8, -60.0019) -> (-8, -150.0019)
  line L2 (-8, -150.0019) -> (8, -150.0019)
  line L3 (8, -150.0019) -> (8, -60.0019)
  line L4 (8, -60.0019) -> (-8, -150.0019) construction
  point P0 (0, -105.0019)
  dimension "d1622" = 105.0019
  dimension "d1623" = 16
  dimension "d1624" = 90
  constraint horizontal L0
  constraint vertical L1
  constraint horizontal L2
  constraint vertical L3
  constraint midpoint L4 P0
  constraint vertical origin P0
  measures "d1622" vertical distance of origin P0
  measures "d1623" horizontal distance of L0.start L0.end
  measures "d1624" vertical distance of L0.end L1.end
extrude "A12 Rear-open cable channel" cut sketch "スケッチ18 (2)" against normal blind 90 bodies 17 in component "Robot V1 - A Holder and Stand"
ref_plane "作業平面1" through (0, 0, 7.71) normal (0, 0, 1) x (1, 0, 0) in component "Robot V1 - B Front Cover"
ref_plane "作業平面2" through (0, 0, 10.11) normal (0, 0, 1) x (1, 0, 0) in component "Robot V1 - B Front Cover"
sketch "スケッチ1 (3)" plane through (0, 0, 7.71) normal (0, 0, 1) x (1, 0, 0) in component "Robot V1 - B Front Cover"
  arc A0 (46, 68) -> (40, 74) centre (40, 68) ccw
  arc A1 (40, 14) -> (46, 20) centre (40, 20) ccw
  arc A2 (-46, 20) -> (-40, 14) centre (-40, 20) ccw
  arc A3 (-40, 74) -> (-46, 68) centre (-40, 68) ccw
  line L0 (-40, 74) -> (40, 74)
  line L1 (46, 68) -> (46, 20)
  line L2 (40, 14) -> (-40, 14)
  line L3 (-46, 20) -> (-46, 68)
  line L4 (40, 68) -> (-40, 20) construction
  point P0 (0, 44)
  dimension "d1631" = 80
  dimension "d1632" = 48
  dimension "d1633" = 6
  dimension "d1634" = 44
  constraint horizontal L0
  constraint horizontal L2
  constraint vertical L3
  constraint vertical L1
  constraint tangent A0 L0
  constraint tangent A0 L1
  constraint tangent A1 L1
  constraint tangent A1 L2
  constraint tangent A2 L2
  constraint tangent A2 L3
  constraint tangent A3 L3
  constraint tangent A3 L0
  constraint equal A0 A1
  constraint equal A0 A2
  constraint equal A0 A3
  constraint midpoint L4 P0
  constraint vertical origin P0
  measures "d1631" horizontal distance of A0.end A3.start
  measures "d1632" vertical distance of A0.start A1.end
  measures "d1633" radius of A0
  measures "d1634" vertical distance of origin P0
extrude "B 01 Head plate" add sketch "スケッチ1 (3)" along normal blind 2.4 separate body makes body 18 in component "Robot V1 - B Front Cover"
sketch "スケッチ2 (3)" plane through (0, 0, 7.71) normal (0, 0, 1) x (1, 0, 0) in component "Robot V1 - B Front Cover"
  arc A0 (41, 16) -> (35, 22) centre (35, 16) ccw
  arc A1 (35, -74) -> (41, -68) centre (35, -68) ccw
  arc A2 (-41, -68) -> (-35, -74) centre (-35, -68) ccw
  arc A3 (-35, 22) -> (-41, 16) centre (-35, 16) ccw
  line L0 (-35, 22) -> (35, 22)
  line L1 (41, 16) -> (41, -68)
  line L2 (35, -74) -> (-35, -74)
  line L3 (-41, -68) -> (-41, 16)
  line L4 (35, 16) -> (-35, -68) construction
  point P0 (0, -26)
  dimension "d1637" = 70
  dimension "d1638" = 84
  dimension "d1639" = 6
  dimension "d1640" = 26
  constraint horizontal L0
  constraint horizontal L2
  constraint vertical L3
  constraint vertical L1
  constraint tangent A0 L0
  constraint tangent A0 L1
  constraint tangent A1 L1
  constraint tangent A1 L2
  constraint tangent A2 L2
  constraint tangent A2 L3
  constraint tangent A3 L3
  constraint tangent A3 L0
  constraint equal A0 A1
  constraint equal A0 A2
  constraint equal A0 A3
  constraint midpoint L4 P0
  constraint vertical origin P0
  measures "d1637" horizontal distance of A0.end A3.start
  measures "d1638" vertical distance of A0.start A1.end
  measures "d1639" radius of A0
  measures "d1640" vertical distance of origin P0
extrude "B 02 Body plate" add sketch "スケッチ2 (3)" along normal blind 2.4 bodies 18 in component "Robot V1 - B Front Cover"
sketch "スケッチ3 (3)" plane through (0, 0, 10.11) normal (0, 0, 1) x (1, 0, 0) in component "Robot V1 - B Front Cover"
  arc A0 (-4, 34) -> (-12, 42) centre (-12, 34) ccw
  arc A1 (-12, 20) -> (-4, 28) centre (-12, 28) ccw
  arc A2 (-24, 28) -> (-16, 20) centre (-16, 28) ccw
  arc A3 (-16, 42) -> (-24, 34) centre (-16, 34) ccw
  line L0 (-16, 42) -> (-12, 42)
  line L1 (-4, 34) -> (-4, 28)
  line L2 (-12, 20) -> (-16, 20)
  line L3 (-24, 28) -> (-24, 34)
  line L4 (-12, 34) -> (-16, 28) construction
  point P0 (-14, 31)
  dimension "d1643" = 4
  dimension "d1644" = 6
  dimension "d1645" = 8
  dimension "d1646" = 14
  dimension "d1647" = 31
  constraint horizontal L0
  constraint horizontal L2
  constraint vertical L3
  constraint vertical L1
  constraint tangent A0 L0
  constraint tangent A0 L1
  constraint tangent A1 L1
  constraint tangent A1 L2
  constraint tangent A2 L2
  constraint tangent A2 L3
  constraint tangent A3 L3
  constraint tangent A3 L0
  constraint equal A0 A1
  constraint equal A0 A2
  constraint equal A0 A3
  constraint midpoint L4 P0
  measures "d1643" horizontal distance of A0.end A3.start
  measures "d1644" vertical distance of A0.start A1.end
  measures "d1645" radius of A0
  measures "d1646" horizontal distance of origin P0
  measures "d1647" vertical distance of origin P0
extrude "B03 Left eye aperture" cut sketch "スケッチ3 (3)" against normal blind 2.4 bodies 18 in component "Robot V1 - B Front Cover"
sketch "スケッチ4 (3)" plane through (0, 0, 10.11) normal (0, 0, 1) x (1, 0, 0) in component "Robot V1 - B Front Cover"
  arc A0 (24, 34) -> (16, 42) centre (16, 34) ccw
  arc A1 (16, 20) -> (24, 28) centre (16, 28) ccw
  arc A2 (4, 28) -> (12, 20) centre (12, 28) ccw
  arc A3 (12, 42) -> (4, 34) centre (12, 34) ccw
  line L0 (12, 42) -> (16, 42)
  line L1 (24, 34) -> (24, 28)
  line L2 (16, 20) -> (12, 20)
  line L3 (4, 28) -> (4, 34)
  line L4 (16, 34) -> (12, 28) construction
  point P0 (14, 31)
  dimension "d1650" = 4
  dimension "d1651" = 6
  dimension "d1652" = 8
  dimension "d1653" = 14
  dimension "d1654" = 31
  constraint horizontal L0
  constraint horizontal L2
  constraint vertical L3
  constraint vertical L1
  constraint tangent A0 L0
  constraint tangent A0 L1
  constraint tangent A1 L1
  constraint tangent A1 L2
  constraint tangent A2 L2
  constraint tangent A2 L3
  constraint tangent A3 L3
  constraint tangent A3 L0
  constraint equal A0 A1
  constraint equal A0 A2
  constraint equal A0 A3
  constraint midpoint L4 P0
  measures "d1650" horizontal distance of A0.end A3.start
  measures "d1651" vertical distance of A0.start A1.end
  measures "d1652" radius of A0
  measures "d1653" horizontal distance of origin P0
  measures "d1654" vertical distance of origin P0
extrude "B03 Right eye aperture" cut sketch "スケッチ4 (3)" against normal blind 2.4 bodies 18 in component "Robot V1 - B Front Cover"
sketch "スケッチ5 (3)" plane through (0, 0, 10.11) normal (0, 0, 1) x (1, 0, 0) in component "Robot V1 - B Front Cover"
  arc A0 (24, 8) -> (21, 11) centre (21, 8) ccw
  arc A1 (21, -17) -> (24, -14) centre (21, -14) ccw
  arc A2 (-24, -14) -> (-21, -17) centre (-21, -14) ccw
  arc A3 (-21, 11) -> (-24, 8) centre (-21, 8) ccw
  line L0 (-21, 11) -> (21, 11)
  line L1 (24, 8) -> (24, -14)
  line L2 (21, -17) -> (-21, -17)
  line L3 (-24, -14) -> (-24, 8)
  line L4 (21, 8) -> (-21, -14) construction
  point P0 (0, -3)
  dimension "d1657" = 42
  dimension "d1658" = 22
  dimension "d1659" = 3
  dimension "d1660" = 3
  constraint horizontal L0
  constraint horizontal L2
  constraint vertical L3
  constraint vertical L1
  constraint tangent A0 L0
  constraint tangent A0 L1
  constraint tangent A1 L1
  constraint tangent A1 L2
  constraint tangent A2 L2
  constraint tangent A2 L3
  constraint tangent A3 L3
  constraint tangent A3 L0
  constraint equal A0 A1
  constraint equal A0 A2
  constraint equal A0 A3
  constraint midpoint L4 P0
  constraint vertical origin P0
  measures "d1657" horizontal distance of A0.end A3.start
  measures "d1658" vertical distance of A0.start A1.end
  measures "d1659" radius of A0
  measures "d1660" vertical distance of origin P0
extrude "B04 Message aperture" cut sketch "スケッチ5 (3)" against normal blind 2.4 bodies 18 in component "Robot V1 - B Front Cover"
sketch "スケッチ6 (3)" plane through (0, 0, 10.11) normal (0, 0, 1) x (1, 0, 0) in component "Robot V1 - B Front Cover"
  circle A0 centre (0, -35) radius 12
  dimension "d1663" = 35
  dimension "d1664" = 24
  constraint vertical origin A0.centre
  measures "d1663" vertical distance of origin A0.centre
  measures "d1664" diameter of A0
extrude "B05 Touch aperture" cut sketch "スケッチ6 (3)" against normal blind 2.4 bodies 18 in component "Robot V1 - B Front Cover"
chamfer "B06 Touch entry bevel - EDIT" distance 1 angle 45 1 edges at (-11.1879, -30.6606, 10.11) on bodies 18 in component "Robot V1 - B Front Cover"